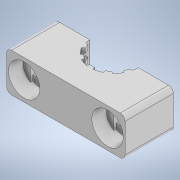
# Autodesk Inventor part: Extruder-Motherboard Cable Clamp
Saved by Autodesk Inventor 2020 (Build 240168000, 168)
## iProperties
Created: 2019-12-23
Part Number: Extruder-Motherboard Cable Clamp
Material: Generic
Document SubType Name: Modeling
Designer: pepd9
Density: 1 g/cm^3
Appearance: Default
Author: pepd9
Autodesk Inventor part; units mm, degrees
ref_plane "YZ Plane" through (0, 0, 0) normal (1, 0, 0) x (0, 1, 0)
ref_plane "XZ Plane" through (0, 0, 0) normal (0, 1, 0) x (-1, 0, 0)
ref_plane "XY Plane" through (0, 0, 0) normal (0, 0, 1) x (1, 0, 0)
sketch "Sketch1" plane through (0, 0, 0) normal (0, 0, 1) x (1, 0, 0)
  circle A0 centre (-3.625, -4) radius 1.7 projected
  arc A1 (-6.25, 0) -> (-7.25, -1) centre (-6.25, -1) ccw projected
  line L0 (-7.25, -1) -> (-7.25, -7) projected
  arc A2 (-7.25, -7) -> (-6.25, -8) centre (-6.25, -7) ccw projected
  line L1 (0, -8) -> (-6.25, -8) projected
  line L2 (0, 0) -> (0, -8) projected
  line L3 (-6.25, 0) -> (0, 0) projected
  circle A3 centre (13.625, -4) radius 1.7 projected
  arc A4 (16.25, -8) -> (17.25, -7) centre (16.25, -7) ccw projected
  line L4 (17.25, -1) -> (17.25, -7) projected
  arc A5 (17.25, -1) -> (16.25, 0) centre (16.25, -1) ccw projected
  line L5 (10, 0) -> (16.25, 0) projected
  line L6 (10, 0) -> (10, -8) projected
  line L7 (16.25, -8) -> (10, -8) projected
  line L8 (0, -8) -> (10, -8)
  line L9 (10, -8) -> (10, 0)
  line L10 (10, 0) -> (0, 0)
  line L11 (0, 0) -> (0, -8)
  constraints: 8 end point, 2 parallel, 1 horizontal, 1 perpendicular
extrude "Extrusion1" add sketch "Sketch1" along normal blind 10 contours A0 | L3 L2 L1 A2 L0 A1 | L10 L6 L8 L2 | L5 A5 L4 A4 L7 L6 | A3
sketch "Sketch2" plane through (-6.25, 0, 0) normal (0, 1, 0) x (1, 0, 0)
  arc A0 (7.7995, 3.6186) -> (6.8051, 2.2897) centre (11.25, 0) ccw projected
  circle A1 centre (11.25, 0) radius 5
  point P0 (6.25, 0)
  constraints: 1 coincident, 3 other
extrude "Extrusion2" cut sketch "Sketch2" against normal through all
sketch "Sketch3" plane through (-6.25, 0, 10) normal (0, 1, 0) x (1, 0, 0)
  line L0 (0, 10) -> (0, 15.75) projected
  line L1 (0, 10) -> (6.25, 10) projected
  arc A0 (6.348, 10.985) -> (6.25, 10) centre (11.25, 10) ccw projected
  line L2 (6.348, 10.985) -> (6.8461, 11.0286) projected
  line L3 (6.8461, 11.0286) -> (7.1881, 11.9683) projected
  line L4 (7.1881, 11.9683) -> (6.8051, 12.2897) projected
  arc A1 (7.7995, 13.6186) -> (6.8051, 12.2897) centre (11.25, 10) ccw projected
  line L5 (7.7995, 13.6186) -> (8.2325, 13.3686) projected
  line L6 (8.2325, 13.3686) -> (9.0517, 13.9421) projected
  line L7 (9.0517, 13.9421) -> (8.9223, 14.4251) projected
  arc A2 (10.499, 14.9433) -> (8.9223, 14.4251) centre (11.25, 10) ccw projected
  line L8 (10.499, 14.9433) -> (10.7104, 14.4901) projected
  line L9 (10.7104, 14.4901) -> (11.7104, 14.4901) projected
  line L10 (11.7104, 14.4901) -> (11.8814, 14.96) projected
  arc A3 (13.4702, 14.48) -> (11.8814, 14.96) centre (11.25, 10) ccw projected
  line L11 (13.4702, 14.48) -> (13.3834, 13.9876) projected
  line L12 (13.3834, 13.9876) -> (14.2025, 13.4141) projected
  line L13 (14.2025, 13.4141) -> (14.6121, 13.7008) projected
  arc A4 (15.6383, 12.3964) -> (14.6121, 13.7008) centre (11.25, 10) ccw projected
  line L14 (15.6383, 12.3964) -> (15.2848, 12.0428) projected
  line L15 (15.2848, 12.0428) -> (15.6268, 11.1031) projected
  line L16 (15.6268, 11.1031) -> (16.1268, 11.1031) projected
  arc A5 (16.25, 10) -> (16.1268, 11.1031) centre (11.25, 10) ccw projected
  line L17 (16.25, 10) -> (22.5, 10) projected
  line L18 (22.5, 15.75) -> (22.5, 10) projected
  arc A6 (6.25, 10) -> (16.25, 10) centre (11.25, 10) ccw projected
  line L19 (16.25, 10) -> (6.25, 10)
  circle A7 centre (11.25, 10) radius 5
  line L20 (6.348, 9.015) -> (6.8461, 8.9714)
  line L21 (6.8461, 8.9714) -> (7.1881, 8.0317)
  line L22 (7.1881, 8.0317) -> (6.8051, 7.7103)
  line L23 (0, 15.75) -> (22.5, 15.75) projected
  constraints: 8 end point, 4 symmetric about line, 1 coincident, 1 horizontal, 3 other
ref_plane "Work Plane1" through (0.098, -1, -2.2897) normal (0, -1, 0) x (1, 0, 0)
extrude "Extrusion3" add sketch "Sketch3" against normal up to surface (1 mm away) contours L20 L21 L22 A6
pattern_circular "Circular Pattern1" count 5 over 140 about axis through (5, 0, 0) along (0, 1, 0) of "Extrusion3"
pattern_linear "Rectangular Pattern1" count 4 spacing 2.3 along (0, -1, 0) of "Extrusion3", "Circular Pattern1"
sketch "Sketch4" plane through (0, 0, 10) normal (0, 0, 1) x (1, 0, 0)
  circle A0 centre (-3.625, -4) radius 1.7 projected
  circle A1 centre (13.625, -4) radius 1.7 projected
  point P0 (0, 0)
hole "Hole1" at (-3.625, -4, 10) at (13.625, -4, 10) direction (0, 0, -1) diameter 3.4 end through all counterbore diameter 6.5 counterbore depth 3 clearance for "Socket Head Cap Screw" size "M3" standard "Ansi Metric M Profile"
sketch "Sketch5" plane through (-3.625, -4, 7) normal (0, 0, 1) x (1, 0, 0)
  circle A0 centre (0, 0) radius 3.25 projected
  circle A1 centre (0, 0) radius 1.7 projected
  circle A2 centre (17.25, 0) radius 3.25 projected
  circle A3 centre (17.25, 0) radius 1.7 projected
  line L0 (-1.7, -3.459) -> (1.7, -3.459)
  line L1 (1.7, -3.459) -> (1.7, 3.459)
  line L2 (1.7, 3.459) -> (-1.7, 3.459)
  line L3 (-1.7, 3.459) -> (-1.7, -3.459)
  line L4 (-1.7, -3.459) -> (1.7, 3.459) construction
  line L5 (1.7, -3.459) -> (-1.7, 3.459) construction
  line L6 (15.55, -3.459) -> (18.95, -3.459)
  line L7 (18.95, -3.459) -> (18.95, 3.459)
  line L8 (18.95, 3.459) -> (15.55, 3.459)
  line L9 (15.55, 3.459) -> (15.55, -3.459)
  line L10 (15.55, -3.459) -> (18.95, 3.459) construction
  line L11 (18.95, -3.459) -> (15.55, 3.459) construction
  point P0 (3.625, 4)
  point P1 (15.55, 0)
  point P2 (15.55, -2.7699)
  point P3 (18.95, -2.7699)
  point P4 (18.95, 0)
  point P5 (15.55, 2.7699)
  point P6 (18.95, 2.7699)
  point P7 (-1.7, 2.7699)
  point P8 (-1.7, 0)
  point P9 (1.7, 0)
  point P10 (1.7, 2.7699)
  point P11 (-1.7, -2.7699)
  point P12 (1.7, -2.7699)
  dimension "d19" = 3.4
  dimension "d20" = 3.4
  constraints: 24 end point, 4 midpoint, 4 parallel, 2 horizontal, 2 perpendicular, 1 point on line
  measures "d19" distance of L2.end L1.end
  measures "d20" distance of L8.end L7.end
extrude "Extrusion4" cut sketch "Sketch5" against normal blind 0.5 contours L1 A1 L3 A0 | A0 L3 A1 L1 | L7 A3 L9 A2 | A2 L9 A3 L7
sketch "Sketch6" plane through (-3.625, -4, 6.5) normal (0, 0, 1) x (1, 0, 0)
  line L0 (-1.7, 0) -> (-1.7, 2.7699) projected
  arc A0 (1.7, 0) -> (-1.7, 0) centre (0, 0) ccw projected
  line L1 (1.7, 2.7699) -> (1.7, 0) projected
  arc A1 (1.7, 2.7699) -> (-1.7, 2.7699) centre (0, 0) ccw projected
  arc A2 (-1.7, -2.7699) -> (1.7, -2.7699) centre (0, 0) ccw projected
  line L2 (1.7, 0) -> (1.7, -2.7699) projected
  arc A3 (-1.7, 0) -> (1.7, 0) centre (0, 0) ccw projected
  line L3 (-1.7, -2.7699) -> (-1.7, 0) projected
  line L4 (18.95, 0) -> (18.95, -2.7699) projected
  arc A4 (15.55, 0) -> (18.95, 0) centre (17.25, 0) ccw projected
  line L5 (15.55, -2.7699) -> (15.55, 0) projected
  arc A5 (15.55, -2.7699) -> (18.95, -2.7699) centre (17.25, 0) ccw projected
  arc A6 (18.95, 0) -> (15.55, 0) centre (17.25, 0) ccw projected
  line L6 (18.95, 2.7699) -> (18.95, 0) projected
  arc A7 (18.95, 2.7699) -> (15.55, 2.7699) centre (17.25, 0) ccw projected
  line L7 (15.55, 0) -> (15.55, 2.7699) projected
  line L8 (-3.4281, -1.7) -> (3.4281, -1.7)
  line L9 (3.4281, -1.7) -> (3.4281, 1.7)
  line L10 (3.4281, 1.7) -> (-3.4281, 1.7)
  line L11 (-3.4281, 1.7) -> (-3.4281, -1.7)
  line L12 (-3.4281, -1.7) -> (3.4281, 1.7) construction
  line L13 (3.4281, -1.7) -> (-3.4281, 1.7) construction
  line L14 (20.0199, -1.7) -> (14.4801, -1.7)
  line L15 (14.4801, -1.7) -> (14.4801, 1.7)
  line L16 (14.4801, 1.7) -> (20.0199, 1.7)
  line L17 (20.0199, 1.7) -> (20.0199, -1.7)
  line L18 (20.0199, -1.7) -> (14.4801, 1.7) construction
  line L19 (14.4801, -1.7) -> (20.0199, 1.7) construction
  point P0 (3.625, 4)
  point P1 (15.55, -1.7)
  point P2 (17.25, -1.7)
  point P3 (18.95, -1.7)
  point P4 (18.95, 1.7)
  point P5 (17.25, 1.7)
  point P6 (15.55, 1.7)
  point P7 (1.7, 1.7)
  point P8 (0, 1.7)
  point P9 (1.7, 0)
  point P10 (1.7, 0)
  point P11 (1.7, 0)
  point P12 (1.7, 0)
  point P13 (-1.7, -1.7)
  point P14 (0, -1.7)
  point P15 (-1.7, 1.7)
  point P16 (1.7, -1.7)
  dimension "d23" = 3.4
  dimension "d24" = 3.4
  constraints: 24 end point, 4 midpoint, 4 parallel, 2 horizontal, 2 perpendicular, 1 point on circle
  measures "d23" distance of L9.end L8.end
  measures "d24" distance of L14.end L15.end
extrude "Extrusion5" cut sketch "Sketch6" against normal blind 0.5 contours L0 L10 A0 | A3 L8 L3 | L10 L1 A0 | A3 L2 L8 | L4 L14 A4 | A6 L16 L6 | L14 L5 A4 | A6 L7 L16
body "Solid1"
